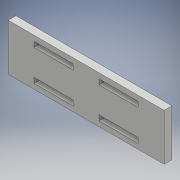
# Autodesk Inventor part: Mounting_base
Saved by Autodesk Inventor 2017 (Build 210142000, 142)
## iProperties
Created: 2017-11-15
Part Number: Mounting_base
Material: Generic
Document SubType Name: Modeling
Designer: julie
Density: 1 g/cm^3
Appearance: Default
Author: julie
Autodesk Inventor part; units mm, degrees
ref_plane "YZ Plane" through (0, 0, 0) normal (1, 0, 0) x (0, 1, 0)
ref_plane "XZ Plane" through (0, 0, 0) normal (0, 1, 0) x (-1, 0, 0)
ref_plane "XY Plane" through (0, 0, 0) normal (0, 0, 1) x (1, 0, 0)
sketch "Sketch1" plane through (0, 0, 0) normal (0, 1, 0) x (-1, 0, 0)
  line L0 (0, 0) -> (-60, 0)
  line L1 (-60, 0) -> (-60, 18)
  line L2 (-60, 18) -> (0, 18)
  line L3 (0, 18) -> (0, 0)
  dimension "d0" = 60
  dimension "d1" = 18
  constraints: 8 end point, 2 parallel, 1 horizontal, 1 perpendicular
  measures "d0" distance of L1.end L2.end
  measures "d1" distance of L0.end L1.end
extrude "Extrusion1" add sketch "Sketch1" along normal blind 3
sketch "Sketch3" plane through (0, 3, 0) normal (0, 1, 0) x (1, 0, 0)
  line L0 (10, -16) -> (25, -16)
  line L1 (25, -16) -> (25, -14)
  line L2 (25, -14) -> (10, -14)
  line L3 (10, -14) -> (10, -16)
  line L4 (10, -2) -> (25, -2)
  line L5 (25, -2) -> (25, -4)
  line L6 (25, -4) -> (10, -4)
  line L7 (10, -4) -> (10, -2)
  line L8 (60, 0) -> (0, 0) projected
  line L9 (0, 0) -> (0, -18) projected
  line L10 (0, -18) -> (60, -18) projected
  line L11 (60, -18) -> (60, 0) projected
  line L12 (30, 6.382) -> (30, -24.5999) construction
  line L13 (50, -16) -> (35, -16)
  line L14 (35, -16) -> (35, -14)
  line L15 (35, -14) -> (50, -14)
  line L16 (50, -14) -> (50, -16)
  line L17 (50, -2) -> (35, -2)
  line L18 (35, -2) -> (35, -4)
  line L19 (35, -4) -> (50, -4)
  line L20 (50, -4) -> (50, -2)
  dimension "d13" = 15
  dimension "d14" = 2
  dimension "d15" = 15
  dimension "d16" = 2
  dimension "d17" = 10
  dimension "d18" = 0
  dimension "d19" = 2
  dimension "d20" = 10
  dimension "d21" = 10
  constraints: 34 end point, 8 symmetric about line, 4 parallel, 3 perpendicular, 2 horizontal
  measures "d13" distance of L2.end L1.end
  measures "d14" distance of L1.end L0.end
  measures "d15" distance of L5.end L6.end
  measures "d16" distance of L4.end L5.end
  measures "d17" distance between parallel lines of L2 L6
  measures "d18" distance between parallel lines of L1 L5
  measures "d19" distance between parallel lines of L10 L0
  measures "d20" distance between parallel lines of L9 L3
  measures "d21" distance between parallel lines of L11 L16
extrude "Extrusion3" cut sketch "Sketch3" against normal through all contours L3 L2 L1 L0 | L4 L5 L6 L7 | L13 L14 L15 L16 | L20 L19 L18 L17
body "Solid1"
